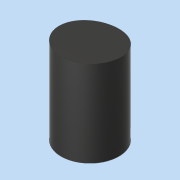
# Autodesk Inventor part: sailScrewCoverCurved
Saved by Autodesk Inventor 2017 (Build 210142000, 142)
## iProperties
Created: 2016-12-18
Part Number: sailScrewCoverCurved
Material: ABS Plastic
Document SubType Name: Modeling
Designer: techn
Density: 1.06 g/cm^3
Appearance: Smooth - Black
Author: techn
Autodesk Inventor part; units mm, degrees
ref_plane "YZ Plane" through (0, 0, 0) normal (1, 0, 0) x (0, 1, 0)
ref_plane "XZ Plane" through (0, 0, 0) normal (0, 1, 0) x (-1, 0, 0)
ref_plane "XY Plane" through (0, 0, 0) normal (0, 0, 1) x (1, 0, 0)
sketch "Sketch1" plane through (0, 0, 0) normal (0, 1, 0) x (-1, 0, 0)
  circle A0 centre (0, 0) radius 3.175
  dimension "d0" = 6.35
  constraints: 1 centre point, 1 coincident
  measures "d0" diameter of A0
extrude "Extrusion1" add sketch "Sketch1" along normal blind 9.525
sketch "Sketch2" plane through (0, 0, 0) normal (1, 0, 0) x (0, 1, 0)
  line L0 (9.525, -3.175) -> (9.525, 3.175) projected
  line L1 (9.525, 3.175) -> (9.525, 0) construction
  line L2 (0, -3.175) -> (9.525, -3.175) projected
  line L3 (9.525, 0) -> (9.0202, -3.175) construction
  spline S0 degree 2 poles (9.525, 3.175) (9.525, 0) (9.0202, -3.175) knots 1 1 1 2 2 2
  point P0 (0, 0)
  constraints: 1 midpoint, 1 point on line, 3 other
extrude "Extrusion2" cut sketch "Sketch2" along normal through all both and the other way through all
body "Solid1"
